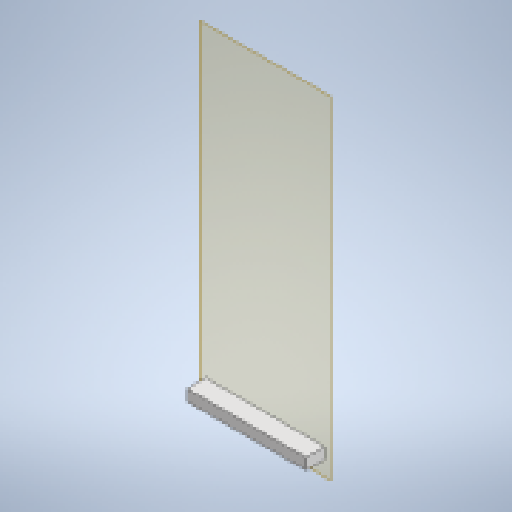
# Autodesk Inventor part: 부품82
Saved by Autodesk Inventor 2024 (Build 280153000, 153)
## iProperties
Created: 2024-09-09
Part Number: 부품82
Material: PMMA 플라스틱
Document SubType Name: Modeling
Designer: Eungang
Density: 1.188 g/cm^3
Appearance: 폴리카보네이트 - 선명
Author: Eungang
Autodesk Inventor part; units mm, degrees
ref_plane "YZ Plane" through (0, 0, 0) normal (1, 0, 0) x (0, 1, 0)
ref_plane "XZ Plane" through (0, 0, 0) normal (0, 1, 0) x (-1, 0, 0)
ref_plane "XY Plane" through (0, 0, 0) normal (0, 0, 1) x (1, 0, 0)
sketch "스케치1" plane through (0, 0, 0.2) normal (0, 0, 1) x (1, 0, 0)
  circle A0 centre (-22.9203, -41.3997) radius 1.35 projected
  circle A1 centre (-22.9203, 35.0003) radius 1.35 projected
  line L0 (-31.9205, -84) -> (-31.9205, 78) projected
  line L1 (31.9205, -84) -> (-31.9205, -84) projected
  line L2 (31.9205, 78) -> (31.9205, -84) projected
  line L3 (-31.9205, 78) -> (31.9205, 78) projected
  circle A2 centre (-22.9203, -75) radius 1.45 projected
  circle A3 centre (-22.9203, 69) radius 1.45 projected
  line L4 (-31.9205, -84) -> (31.9205, -84)
  line L5 (31.9205, -84) -> (31.9205, -78)
  line L6 (31.9205, -78) -> (-31.9205, -78)
  line L7 (-31.9205, -78) -> (-31.9205, -84)
  point P0 (0, 0)
  point P1 (-31.9205, -78)
  constraints: 8 end point, 2 parallel, 1 horizontal, 1 perpendicular, 1 point on line
extrude "돌출1" add sketch "스케치1" along normal blind 136.628 contours L0 L6 L2 L1
sketch "스케치4" plane through (-31.9205, -84, 0.2) normal (0, -1, 0) x (1, 0, 0)
  circle A0 centre (2.641, 9) radius 1.35 projected
  circle A1 centre (2.641, 75.2636) radius 1.35 projected
  point P0 (31.9205, -0.2)
extrude "돌출4" cut sketch "스케치4" against normal through all contours A1
sketch "스케치5" plane through (-31.9205, -84, 0.2) normal (0, -1, 0) x (1, 0, 0)
  circle A0 centre (2.641, 127.428) radius 1.35 projected
  point P0 (31.9205, -0.2)
extrude "돌출5" cut sketch "스케치5" against normal up to next
sketch "스케치6" plane through (-31.9205, -78, 0.2) normal (0, 1, 0) x (1, 0, 0)
  circle A0 centre (2.241, -9) radius 1.35 projected
  point P0 (31.9205, 0.2)
extrude "돌출6" cut sketch "스케치6" against normal up to next
